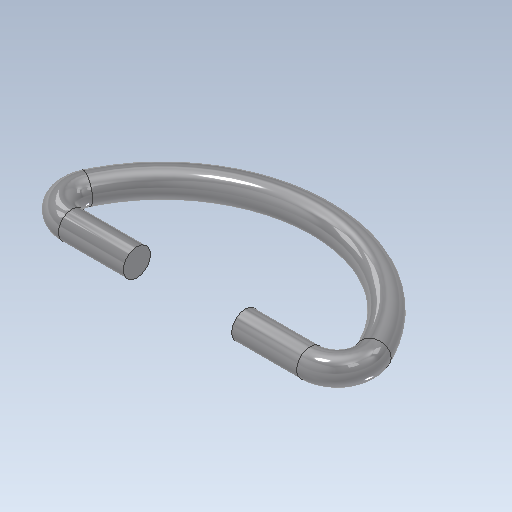
# Autodesk Inventor part: Thumb Screw Handle
Saved by Autodesk Inventor 2020 (Build 240168000, 168)
## iProperties
Created: 2012-10-13
Part Number: Thumb Screw Handle
Material: Steel, Mild
Document SubType Name: Modeling
Designer: Lance
Mass: 2.1284 g
Surface Area: 4.43631 cm^2
Volume: 0.271133 cm^3
Density: 7.85 g/cm^3
Appearance: Aluminum - Polished
Author: Lance
Autodesk Inventor part; units mm, degrees
ref_plane "YZ Plane" through (0, 0, 0) normal (1, 0, 0) x (0, 1, 0)
ref_plane "XZ Plane" through (0, 0, 0) normal (0, 1, 0) x (-1, 0, 0)
ref_plane "XY Plane" through (0, 0, 0) normal (0, 0, 1) x (1, 0, 0)
sketch "Sketch1" plane through (0, 0, 0) normal (1, 0, 0) x (0, 1, 0)
  circle A0 centre (0, 0) radius 1.25
  dimension "d0" = 2.5
  constraints: 1 centre point, 1 coincident
  measures "d0" diameter of A0
sketch "Sketch2" plane through (0, 0, 0) normal (0, 1, 0) x (-1, 0, 0)
  line L0 (0, -14.9286) -> (0, 5.5714) projected
  arc A0 (13.2647, -3.5588) -> (11, 0) centre (11, -2.5) ccw
  arc A1 (-11, 0) -> (-13.2647, -3.5588) centre (-11, -2.5) ccw
  line L1 (11, 0) -> (-11, 0)
  arc A2 (-13.2647, -3.5588) -> (13.2647, -3.5588) centre (0, 2.6429) ccw
  point P0 (0, 0)
  dimension "d4" = 5
  dimension "d5" = 27
  dimension "d6" = 12
  constraints: 6 point on circle, 4 tangent, 3 centre point, 2 end point, 1 midpoint, 1 other
  measures "d4" diameter of A0
  measures "d6" distance edge to line of A2 L1
sweep "Sweep1" add profiles "Sketch1" path "Sketch2" path curves L1 A1 A2 A0
sketch "Sketch3" plane through (0, 0, 0) normal (0, 1, 0) x (-1, 0, 0)
  line L0 (5, -1.25) -> (-5, -1.25)
  line L1 (-5, -1.25) -> (-5, 1.25)
  line L2 (-5, 1.25) -> (5, 1.25)
  line L3 (5, 1.25) -> (5, -1.25)
  line L4 (11, 1.25) -> (-11, 1.25) projected
  line L5 (11, -1.25) -> (-11, -1.25) projected
  point P0 (0, 0)
  point P1 (0, 1.25)
  dimension "d8" = 10
  constraints: 8 end point, 2 collinear, 2 parallel, 1 horizontal, 1 midpoint, 1 perpendicular, 1 vertical alignment
  measures "d8" distance between parallel lines of L1 L3
extrude "Extrusion1" cut sketch "Sketch3" along normal through all both and the other way through all
body "Solid1"
